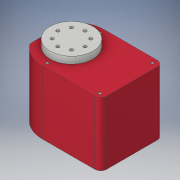
# Autodesk Inventor part: servo
Saved by Autodesk Inventor 2019 (Build 230136000, 136)
## iProperties
Created: 2019-02-02
Part Number: servo
Material: Aluminum
Document SubType Name: Modeling
Designer: suchanek
Density: 2.7 g/cm^3
Appearance: Satin
Author: suchanek
Autodesk Inventor part; units mm, degrees
ref_plane "YZ Plane" through (0, 0, 0) normal (1, 0, 0) x (0, 1, 0)
ref_plane "XZ Plane" through (0, 0, 0) normal (0, 1, 0) x (-1, 0, 0)
ref_plane "XY Plane" through (0, 0, 0) normal (0, 0, 1) x (1, 0, 0)
sketch "Sketch1" plane through (0, 0, 0) normal (0, 1, 0) x (-1, 0, 0)
  line L0 (21.5, 16) -> (8.5, 16)
  line L1 (-21.5, 16) -> (-21.5, -16)
  line L2 (-21.5, -16) -> (8.5, -16)
  line L3 (21.5, -16) -> (21.5, 16)
  line L4 (21.5, 16) -> (-21.5, -16) construction
  line L5 (-21.5, 16) -> (21.5, -16) construction
  line L6 (8.5, 16) -> (8.5, -16)
  line L7 (8.5, 16) -> (-21.5, 16)
  line L8 (8.5, -16) -> (21.5, -16)
  arc A0 (21.5, 9.3274) -> (8.5, 16) centre (8.5, 0) ccw
  arc A1 (8.5, -16) -> (21.5, -9.3274) centre (8.5, 0) ccw
  point P0 (0, 0)
  dimension "d0" = 43
  dimension "d1" = 32
  dimension "d8" = 30
  dimension "d9" = 16
  dimension "d10" = 16
  constraints: 18 end point, 5 parallel, 4 point on circle, 2 centre point, 2 horizontal, 2 midpoint, 2 perpendicular, 2 point on line, 2 tangent, 1 vertical, 1 vertical alignment
  measures "d0" distance of L0.start L1.start
  measures "d1" distance of L3.start L0.start
  measures "d8" distance between parallel lines of L1 L6
  measures "d9" radius of A0
  measures "d10" radius of A1
extrude "Extrusion1" add sketch "Sketch1" along normal blind 32.5 contours A0 L3 A1 L6 | L6 L2 L1 L7
sketch "Sketch2" plane through (0, 32.5, 0) normal (0, 1, 0) x (1, 0, 0)
  circle A0 centre (-9.5, 0) radius 11
  line L0 (21.5, -16) -> (21.5, 16) projected
  line L1 (-8.5, -16) -> (21.5, -16) projected
  point P0 (0, 0)
  dimension "d4" = 31
  dimension "d5" = 22
  dimension "d28" = 16
  constraints: 1 centre point
  measures "d4" distance from line of L0 A0.centre
  measures "d5" diameter of A0
  measures "d28" distance from line of L1 A0.centre
extrude "Extrusion2" add sketch "Sketch2" along normal blind 3.5
fillet "Fillet1" radius 3 4 edges at (-21.5, 16.25, 9.3274) (-21.5, 16.25, -9.3274) (21.5, 16.25, -16) (21.5, 16.25, 16)
sketch "Sketch3" plane through (-9.5, 36, 0) normal (0, 1, 0) x (1, 0, 0)
  circle A0 centre (-7, 0) radius 0.8
  circle A1 centre (0, 0) radius 11 projected
  circle A2 centre (-4.9497, -4.9497) radius 0.8
  circle A3 centre (0, -7) radius 0.8
  circle A4 centre (4.9497, -4.9497) radius 0.8
  circle A5 centre (7, 0) radius 0.8
  circle A6 centre (4.9497, 4.9497) radius 0.8
  circle A7 centre (0, 7) radius 0.8
  circle A8 centre (-4.9497, 4.9497) radius 0.8
  point P0 (9.5, 0)
  dimension "d12" = 1.6
  dimension "d14" = 7
  dimension "d17" = 360
  constraints: 8 centre point, 1 coincident, 1 horizontal alignment, 17 other
  measures "d12" diameter of A0
  measures "d14" distance of A1.centre A0.centre
extrude "Extrusion3" cut sketch "Sketch3" against normal up to surface (3.5 mm away) contours A0 | A2 | A3 | A4 | A5 | A6 | A7 | A8
sketch "Sketch4" plane through (0, 32.5, 0) normal (0, 1, 0) x (1, 0, 0)
  circle A0 centre (-8.5, -13.5) radius 0.7
  circle A1 centre (18.5, -13.5) radius 0.7
  circle A2 centre (18.5, 13.5) radius 0.7
  circle A3 centre (-8.5, 13.5) radius 0.7
  line L0 (-8.5, -16) -> (18.5, -16) projected
  line L1 (21.5, -13) -> (21.5, 13) projected
  point P0 (0, 0)
  dimension "d21" = 1.4
  dimension "d22" = 27
  dimension "d23" = 2.5
  dimension "d24" = 3
  dimension "d25" = 27
  constraints: 4 centre point, 3 equal radius, 2 horizontal alignment, 2 vertical alignment
  measures "d21" diameter of A3
  measures "d22" distance of A1.centre A2.centre
  measures "d23" distance from line of A1.centre L0
  measures "d24" distance from line of L1 A1.centre
  measures "d25" distance of A1.centre A0.centre
extrude "Extrusion4" cut sketch "Sketch4" against normal through all
body "Solid1"
